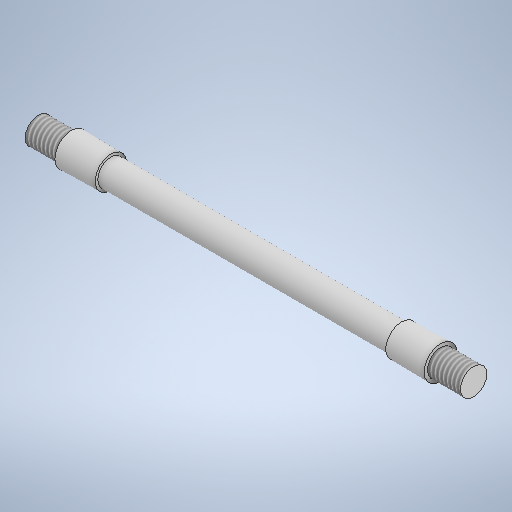
# Autodesk Inventor part: Schwarnenhals
Saved by Autodesk Inventor 2025.1 (Build 291241000, 241)
## iProperties
Created: 2025-01-26
Part Number: Schwarnenhals
Material: Generisch
Document SubType Name: Modeling
Designer: joebe
Density: 1 g/cm^3
Appearance: Vorgabe
Author: joebe
Autodesk Inventor part; units mm, degrees
ref_plane "YZ Plane" through (0, 0, 0) normal (1, 0, 0) x (0, 1, 0)
ref_plane "XZ Plane" through (0, 0, 0) normal (0, 1, 0) x (-1, 0, 0)
ref_plane "XY Plane" through (0, 0, 0) normal (0, 0, 1) x (1, 0, 0)
sketch "Skizze1" plane through (0, 0, 0) normal (0, 0, 1) x (1, 0, 0)
  line L0 (0, 5) -> (-11.8602, 4.793)
  line L1 (-12, 4) -> (-100, 4)
  line L2 (-100, 4) -> (-100, 0)
  line L3 (0, 5) -> (0, 4)
  line L4 (0, 4) -> (10, 4)
  line L5 (10, 4) -> (10, 0)
  line L6 (-100, 0) -> (10, 0)
  line L7 (-12, 4) -> (-11.8602, 4.793)
  line L8 (-100, 4) -> (-100, 4.793)
  line L9 (-100, 4.793) -> (-112, 5)
  line L10 (-112, 5) -> (-112, 4)
  line L11 (-112, 4) -> (-122, 4)
  line L12 (-122, 4) -> (-122, 0)
  line L13 (-122, 0) -> (-100, 0)
  point P0 (0, 0)
  dimension "d0" = 8
  dimension "d2" = 10
  dimension "d3" = 10
  dimension "d4" = 12
  dimension "d5" = 8
  dimension "d6" = 1
  dimension "d7" = 100
  dimension "d8" = 100
  dimension "d12" = 12
  dimension "d13" = 10
  constraints: 28 end point, 6 perpendicular, 4 horizontal alignment, 1 horizontal, 1 parallel, 1 point on line, 1 vertical, 1 vertical alignment
  measures "d0" diameter of L4 L6
  measures "d2" diameter of L0.start L6
  measures "d3" distance of L3.end L4.end
  measures "d4" distance of L1.start L3.end
  measures "d5" diameter of L1 L6
  measures "d6" angle of L1 L0
  measures "d7" distance from line of L2 point (0, 0)
  measures "d8" angle of L1 L7
  measures "d12" distance of L10.end L1.end
  measures "d13" distance of L10.end L11.end
revolve "Umdrehung1" add sketch "Skizze1" angle 360 about axis through (-100, 0, 0) along (1, 0, 0)
thread "Gewinde1" size "M8x1.25" class "6g" standard "ISO Metric profile" full length
equation "\"d12\" = d4"
equation "\"d13\" = d3"
